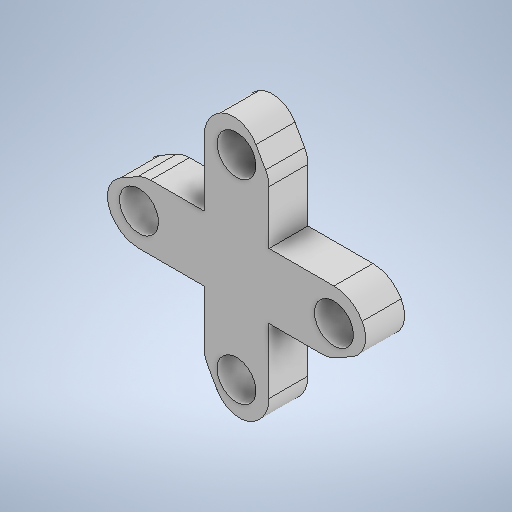
# Autodesk Inventor part: ModuleConnector_Center_Axis
Saved by Autodesk Inventor 2025.1 (Build 291241020, 241B)
## iProperties
Created: 2024-10-06
Part Number: ModuleConnector_Center_Axis
Material: 일반
Document SubType Name: Modeling
Designer: SEON06
Density: 1 g/cm^3
Appearance: 기본값
Author: SEON06
Autodesk Inventor part; units mm, degrees
ref_plane "YZ Plane" through (0, 0, 0) normal (1, 0, 0) x (0, 1, 0)
ref_plane "XZ Plane" through (0, 0, 0) normal (0, 1, 0) x (-1, 0, 0)
ref_plane "XY Plane" through (0, 0, 0) normal (0, 0, 1) x (1, 0, 0)
sketch "스케치1" plane through (0, 0, 0) normal (0, 0, 1) x (1, 0, 0)
  circle A0 centre (0, 0) radius 10
  arc A1 (-2.5, 0) -> (2.5, 0) centre (0, 0) ccw
  arc A2 (2.5, 7.5) -> (-2.5, 7.5) centre (0, 7.5) ccw
  line L0 (-2.5, 7.5) -> (-2.5, 0)
  line L1 (2.5, 7.5) -> (2.5, 0)
  arc A3 (-7.5, 2.5) -> (-7.5, -2.5) centre (-7.5, 0) ccw
  line L2 (-7.5, 2.5) -> (0, 2.5)
  line L3 (-7.5, -2.5) -> (0, -2.5)
  arc A4 (0, -2.5) -> (0, 2.5) centre (0, 0) ccw
  arc A5 (-2.5, -7.5) -> (2.5, -7.5) centre (0, -7.5) ccw
  line L4 (-2.5, -7.5) -> (-2.5, 0)
  line L5 (2.5, -7.5) -> (2.5, 0)
  arc A6 (2.5, 0) -> (-2.5, 0) centre (0, 0) ccw
  arc A7 (7.5, -2.5) -> (7.5, 2.5) centre (7.5, 0) ccw
  line L6 (7.5, -2.5) -> (0, -2.5)
  line L7 (7.5, 2.5) -> (0, 2.5)
  arc A8 (0, 2.5) -> (0, -2.5) centre (0, 0) ccw
  point P0 (-2.5, 2.5)
  point P1 (-2.5, -2.5)
  point P2 (2.5, -2.5)
  point P3 (2.5, 2.5)
  dimension "d0" = 20
  dimension "d1" = 5
  dimension "d2" = 5
  dimension "d5" = 360
  constraints: 16 end point, 16 point on circle, 9 centre point, 3 tangent, 2 coincident, 2 vertical, 1 vertical alignment, 41 other
  measures "d0" diameter of A0
  measures "d1" diameter of A1
  measures "d2" diameter of A2
extrude "돌출1" add sketch "스케치1" along normal blind 3 contours A7 L6 L5 L1 L7 | A2 L1 L7 L2 L0 | A5 L4 L3 L6 L5 | A3 L2 L0 L4 L3 | L6 A1 L5 | L1 A4 L7 | L2 A6 L0 | L4 A1 L3 | A1 A6 A4
sketch "스케치2" plane through (0, 0, 3) normal (0, 0, 1) x (1, 0, 0)
  arc A0 (2.5, 7.5) -> (-2.5, 7.5) centre (0, 7.5) ccw projected
  circle A1 centre (0, 7.5) radius 1.5
  point P0 (0, 0)
  dimension "d9" = 3
  constraints: 1 centre point, 1 coincident
  measures "d9" diameter of A1
extrude "돌출2" cut sketch "스케치2" against normal through all
pattern_circular "원형 패턴1" count 4 over 360 about axis through (0, 0, -10) along (0, 0, 1) of "돌출2"
sketch "스케치3" plane through (0, 0, 3) normal (0, 0, 1) x (1, 0, 0)
  arc A0 (2.5, 7.5) -> (-2.5, 7.5) centre (0, 7.5) ccw projected
  line L0 (1, 9.7913) -> (2.5, 7.1456)
  line L1 (2.5, 2.5) -> (2.5, 7.5) projected
  circle A1 centre (0, 7.5) radius 1.5 projected
  point P0 (0, 0)
  dimension "d15" = 0.5
  dimension "d16" = 1
  constraints: 2 end point, 1 point on circle, 1 point on line
  measures "d15" distance edge to line of A1 L0
  measures "d16" horizontal distance of L0.start A0.centre
extrude "돌출3" cut sketch "스케치3" against normal through all contours L1 L0 A0
fillet "모깎기1" radius 2 1 edges at (1, 9.7913, 1.5)
fillet "모깎기2" radius 2 1 edges at (2.5, 7.1456, 1.5)
pattern_circular "원형 패턴2" count 4 over 360 about axis through (0, 0, -10) along (0, 0, 1) of "돌출3", "모깎기1", "모깎기2"
equation "\"d1\" = 0.25 * d0"
equation "\"d2\" = d1"
